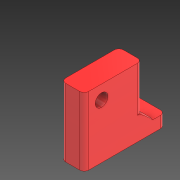
# Autodesk Inventor part: CH_01_0039_kradex_mount_1
Saved by Autodesk Inventor 2022 (Build 260153000, 153)
## iProperties
Created: 2022-05-23
Part Number: CH_01_0039_kradex_mount_1
Material: Generic
Document SubType Name: Modeling
Designer: Tomasz Krakowski
Density: 1 g/cm^3
Appearance: Light Red
Author: Tomasz Krakowski
Autodesk Inventor part; units mm, degrees
ref_plane "YZ Plane" through (0, 0, 0) normal (1, 0, 0) x (0, 1, 0)
ref_plane "XZ Plane" through (0, 0, 0) normal (0, 1, 0) x (-1, 0, 0)
ref_plane "XY Plane" through (0, 0, 0) normal (0, 0, 1) x (1, 0, 0)
sketch "Sketch1" plane through (0, 0, 0) normal (0, 1, 0) x (-1, 0, 0)
  line L0 (0, 0) -> (20, 0)
  line L1 (20, 0) -> (20, -10)
  line L2 (20, -10) -> (-10, -10)
  line L3 (-10, -10) -> (-10, 25)
  line L4 (-10, 25) -> (0, 25)
  line L5 (0, 25) -> (0, 0)
  dimension "d0" = 10
  dimension "d1" = 25
  dimension "d2" = 10
  dimension "d3" = 20
  constraints: 12 end point, 5 perpendicular, 1 horizontal
  measures "d0" distance of L0.end L1.end
  measures "d1" distance between parallel lines of L0 L4
  measures "d2" distance between parallel lines of L5 L3
  measures "d3" distance from line of L0.start L1
extrude "Extrusion1" add sketch "Sketch1" along normal blind 5
sketch "Sketch2" plane through (0, 5, 0) normal (0, 1, 0) x (1, 0, 0)
  line L0 (-20, 10) -> (-20, 0) projected
  line L1 (-20, 5) -> (-3, 5) construction
  point P0 (0, 0)
  point P1 (-15, 5)
  dimension "d6" = 5
  dimension "d7" = 12
  constraints: 2 end point, 1 coincident, 1 horizontal, 1 midpoint, 1 point on line
  measures "d6" distance from line of L0 point (-15, 5)
  measures "d7" distance of point (-3, 5) point (-15, 5)
hole "Hole1" at (-3, 5, -5) at (-15, 5, -5) direction (0, -1, 0) diameter 3.5 end through all counterbore diameter 5.5 counterbore depth 3.5
sketch "Sketch3" plane through (0, 5, 0) normal (0, 1, 0) x (1, 0, 0)
  line L0 (0, -25) -> (10, -25) projected
  line L1 (10, -25) -> (10, 10) construction
  line L2 (0, -25) -> (10, -25)
  line L3 (10, -25) -> (10, 0)
  line L4 (10, 0) -> (0, 0)
  line L5 (0, 0) -> (0, -25)
  constraints: 8 end point, 2 parallel, 1 coincident, 1 horizontal, 1 perpendicular, 1 point on line
extrude "Extrusion2" add sketch "Sketch3" along normal blind 24.5
fillet "Fillet1" radius 1 1 edges at (0, 2.5, 0)
fillet "Fillet2" radius 2 7 edges at (-20, 2.5, 0) (0, 14.75, 25) (-20, 2.5, -10) (0, 17.25, 0) (10, 17.25, 0) (10, 2.5, -10) (10, 14.75, 25)
sketch "Sketch4" plane through (0, 0, 1) normal (-1, 0, 0) x (0, 0, 1)
  line L0 (-1, 0) -> (-3, 0) projected
  line L1 (-4.25, 0) -> (-7.75, 0) construction
  point P0 (16.5, 23.5)
  point P1 (-6, 0)
  dimension "d19" = 23.5
  dimension "d20" = 22.5
  constraints: 1 midpoint
  measures "d19" distance from line of point (16.5, 23.5) L0
  measures "d20" horizontal distance of point (16.5, 23.5) point (-6, 0)
hole "Hole2" at (0, 23.5, 17.5) direction (1, 0, 0) diameter 5.5 end through all
chamfer "Chamfer1" distance 5 angle 45 3 edges at (5, 5, 0) (9.4142, 5, 0.5858) (0.5858, 5, 0.5858)
body "Solid1"
